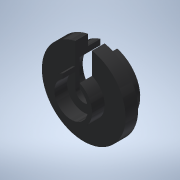
# Autodesk Inventor part: shocks_end
Saved by Autodesk Inventor 2020 (Build 240168000, 168)
## iProperties
Created: 2015-12-04
Part Number: shocks_end
Material: Goma
Document SubType Name: Modeling
Designer: MIGUEL ANGEL
Density: 0.93 g/cm^3
Appearance: Goma - Negro - Versión 1.1
Author: MIGUEL ANGEL
Autodesk Inventor part; units mm, degrees
ref_plane "YZ Plane" through (0, 0, 0) normal (1, 0, 0) x (0, 1, 0)
ref_plane "XZ Plane" through (0, 0, 0) normal (0, 1, 0) x (-1, 0, 0)
ref_plane "XY Plane" through (0, 0, 0) normal (0, 0, 1) x (1, 0, 0)
sketch "Boceto1" plane through (0, 0, 0) normal (0, 1, 0) x (-1, 0, 0)
  circle A0 centre (0, 0) radius 10
  dimension "d3" = 20
  constraints: 1 centre point
  measures "d3" diameter of A0
extrude "Extrusión1" add sketch "Boceto1" along normal blind 6
sketch "Boceto2" plane through (0, 6, 0) normal (0, 1, 0) x (1, 0, 0)
  circle A0 centre (0, 0) radius 20
  dimension "d6" = 40
  constraints: 1 centre point, 1 coincident
  measures "d6" diameter of A0
extrude "Extrusión2" add sketch "Boceto2" along normal blind 6
sketch "Boceto3" plane through (0, 12, 0) normal (0, 1, 0) x (1, 0, 0)
  circle A0 centre (0, 0) radius 15
  dimension "d9" = 30
  constraints: 1 centre point, 1 coincident
  measures "d9" diameter of A0
extrude "Extrusión3" add sketch "Boceto3" along normal blind 6
sketch "Boceto4" plane through (0, 18, 0) normal (0, 1, 0) x (1, 0, 0)
  circle A0 centre (0, 0) radius 4
  circle A1 centre (0, 0) radius 20 projected
  line L0 (-4, 0) -> (-4, -19.5959)
  line L1 (4, 0) -> (4, -19.5959)
  dimension "d12" = 8
  constraints: 4 end point, 4 point on circle, 1 centre point, 1 coincident, 1 parallel, 1 tangent, 1 vertical
  measures "d12" diameter of A0
extrude "Extrusión4" cut sketch "Boceto4" against normal through all contours A0 | L1 A1 L0 A0 picked at (0.1607, -14.6269)
sketch "Boceto5" plane through (0, 18, 0) normal (0, 1, 0) x (1, 0, 0)
  circle A0 centre (0, 0) radius 12.5
  dimension "d15" = 25
  constraints: 1 centre point, 1 coincident
  measures "d15" diameter of A0
extrude "Extrusión5" cut sketch "Boceto5" against normal blind 10
sketch "Boceto6" plane through (0, 0, 0) normal (0, -1, 0) x (1, 0, 0)
  circle A0 centre (0, 0) radius 8
  dimension "d18" = 16
  constraints: 1 centre point, 1 coincident
  measures "d18" diameter of A0
extrude "Extrusión6" cut sketch "Boceto6" against normal up to surface (6 mm away)
